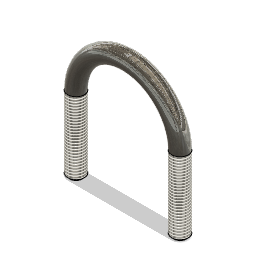
0.883.0500 - Etrier de 10x61x70 - VZC 21400_17 Rep. 75 (Autodesk Fusion 360 design; units mm, degrees)
Autodesk Fusion 360 part; units mm, degrees
note: some values were not read from the file. Chosen so that the rebuilt part matches the saved one: which face or edge a step refers to; how an offset face is resized.
sketch "Sketch1" plane through (0, 0, 0) normal (0, 0, 1) x (1, 0, 0)
  line L0 (0, 0) -> (-100, 0) construction
  line L1 (0, 0) -> (100, 0) construction
  line L2 (0, 0) -> (0, 100) construction
  line L3 (0, 0) -> (0, -100) construction
  circle A0 centre (0, 24.5) radius 24.5 construction
  line L4 (30.5, 0) -> (30.5, -100) construction
  line L5 (30.5, 0) -> (30.5, 100) construction
  line L6 (-30.5, 0) -> (-30.5, -100) construction
  line L7 (-30.5, 0) -> (-30.5, 100) construction
  line L8 (0, 49) -> (0, 54) construction
  line L9 (25.5, 0) -> (25.5, 23.5)
  line L10 (-25.5, 0) -> (-25.5, 23.5)
  line L11 (0, 49) -> (0, 49)
  line L12 (0, 49) -> (0, 49)
  arc A1 (0, 49) -> (-25.5, 23.5) centre (0, 23.5) ccw
  arc A2 (25.5, 23.5) -> (0, 49) centre (0, 23.5) ccw
  line L13 (-25.5, 0) -> (-25.5, -20)
  line L14 (25.5, 0) -> (25.5, -20)
  dimension "d5" = 49
  dimension "d6" = 30.5
  dimension "d7" = 30.5
  dimension "d11" = 25.5
  dimension "d12" = 25.5
  dimension "d13" = 20
  dimension "d14" = 20
  constraint coincident L0.start L1.start
  constraint horizontal L1
  constraint horizontal L0
  constraint vertical L3
  constraint vertical L2
  constraint coincident L0.start A0
  constraint coincident L2 L8.start
  constraint coincident A0 L8.start
  constraint parallel L2 L9
  constraint parallel L2 L10
  constraint tangent L10 A1
  constraint tangent L9 A2
  measures "d5" diameter of A0
  measures "d11" radius of A1
  measures "d12" radius of A2
  measures "d13" distance of L10.start L13.end
  measures "d14" distance of L9.start L14.end
sketch "Sketch2" plane through (0, 0, 0) normal (1, 0, 0) x (0, 0, -1)
  circle A0 centre (0, 54) radius 5
  point P0 (0, 49)
  dimension "d15" = 10
  constraint coincident P0 A0
  measures "d15" diameter of A0
sweep "Sweep1" add profiles "Sketch2" path "Sketch1" along L14 L9 A2 A1 L10 L13 section 1
chamfer "Chamfer1" distance 1.5 angle 45 2 edges at (-32.3081, -20, 4.6616) (28.6919, -20, 4.6616)
thread "Thread1" "ISO Metric profile 10.0 M10x1.5 6g" major diameter 9.85 minor diameter 8.141 pitch 1.5 angle 60 resizes the face on face at (-30.0022, -4.5, -4.9752)
thread "Thread2" "ISO Metric profile 10.0 M10x1.5 6g"
